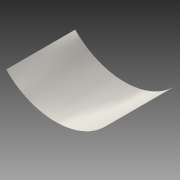
# Autodesk Inventor part: lamina-inox
Saved by Autodesk Inventor 2015 (Build 190159000, 159)
## iProperties
Created: 2016-02-19
Part Number: lamina-inox
Material: Generic
Document SubType Name: Modeling
Designer: al131100X
Density: 1 g/cm^3
Appearance: Default
Author: al131100X
Autodesk Inventor part; units mm, degrees
ref_plane "YZ Plane" through (0, 0, 0) normal (1, 0, 0) x (0, 1, 0)
ref_plane "XZ Plane" through (0, 0, 0) normal (0, 1, 0) x (-1, 0, 0)
ref_plane "XY Plane" through (0, 0, 0) normal (0, 0, 1) x (1, 0, 0)
sketch "Sketch1" plane through (0, 0, 0) normal (0, 1, 0) x (-1, 0, 0)
  arc A0 (2079.7738, 263.7021) -> (3881.891, 268.3125) centre (2978.5428, 1160.9837) ccw
  arc A1 (2080.8354, 264.7618) -> (3880.8295, 269.3723) centre (2978.5428, 1160.9837) ccw
  line L0 (3881.891, 268.3125) -> (3880.8295, 269.3723)
  line L1 (2079.7738, 263.7021) -> (2080.8354, 264.7618)
  point P0 (0, 0)
  dimension "d9" = 1.5
  dimension "d16" = 1800
  dimension "d22" = 1270
  constraints: 4 end point, 4 point on circle, 2 centre point, 1 other
  measures "d9" radial gap between concentric circles of A0 A1
  measures "d16" distance of L0.end L1.end
  measures "d22" radius of A0
extrude "Extrusion1" add sketch "Sketch1" along normal blind 1260
body "Solid1"
